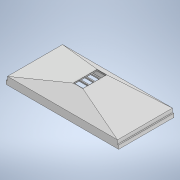
# Autodesk Inventor part: lejek
Saved by Autodesk Inventor 2020.3 (Build 243373000, 373)
## iProperties
Created: 2021-01-13
Part Number: lejek
Material: Ogólny
Document SubType Name: Modeling
Designer: sitar
Density: 1 g/cm^3
Appearance: Domyślna
Author: sitar
Autodesk Inventor part; units mm, degrees
ref_plane "YZ Plane" through (0, 0, 0) normal (1, 0, 0) x (0, 1, 0)
ref_plane "XY Plane" through (0, 0, 0) normal (0, 0, 1) x (1, 0, 0)
sketch "Szkic1" plane through (0, 0, 0) normal (0, 1, 0) x (-1, 0, 0)
  line L0 (57.6, -28.8) -> (-57.6, -28.8)
  line L1 (-57.6, -28.8) -> (-57.6, 28.8)
  line L2 (-57.6, 28.8) -> (57.6, 28.8)
  line L3 (57.6, 28.8) -> (57.6, -28.8)
  line L4 (57.6, -28.8) -> (-57.6, 28.8) construction
  line L5 (-57.6, -28.8) -> (57.6, 28.8) construction
  point P0 (0, 0)
  dimension "d0" = 115.2
  dimension "d1" = 57.6
  constraints: 12 end point, 2 midpoint, 2 parallel, 1 horizontal, 1 perpendicular
  measures "d0" distance of L1.end L2.end
  measures "d1" distance of L0.end L1.end
ref_plane "Płaszczyzna konstrukcyjna3" through (0, 12, 0) normal (0, 1, 0) x (-1, 0, 0)
sketch "Szkic11" plane through (0, 12, 0) normal (0, 1, 0) x (-1, 0, 0)
  line L0 (-5, -12.5) -> (5, -12.5)
  line L1 (5, -12.5) -> (5, 12.5)
  line L2 (5, 12.5) -> (-5, 12.5)
  line L3 (-5, 12.5) -> (-5, -12.5)
  line L4 (-5, -12.5) -> (5, 12.5) construction
  line L5 (5, -12.5) -> (-5, 12.5) construction
  point P0 (0, 0)
  dimension "d41" = 10
  dimension "d42" = 25
  constraints: 12 end point, 2 midpoint, 2 parallel, 1 horizontal, 1 perpendicular
  measures "d41" distance of L2.end L1.end
  measures "d42" distance of L1.end L0.end
loft "Wyciągnięcie złożone3" add profiles "Szkic11", "Szkic1"
shell "Skorupa3" thickness 1.2 removed faces 1 at (-19.2, 0, 9.6)
sketch "Szkic12" plane through (-4.8649, 10.8, -12.1059) normal (0, -1, 0) x (1, 0, 0)
  line L0 (0, 0) -> (0, 24.2118) projected
  line L1 (9.7297, 0) -> (57.0697, -14.67) projected
  line L2 (0, 24.2118) -> (9.7297, 24.2118)
  line L3 (9.7297, 24.2118) -> (9.7297, 0)
  line L4 (9.7297, 0) -> (0, 0)
  line L5 (0, 0) -> (0, 24.2118)
  point P0 (4.8649, 12.1059)
  constraints: 8 end point, 2 parallel, 1 horizontal, 1 perpendicular
extrude "Wyciągnięcie proste7" cut sketch "Szkic12" against normal blind 10
sketch "Szkic13" plane through (-57.6, 0, -28.8) normal (0, -1, 0) x (1, 0, 0)
  line L0 (115.2, 57.6) -> (115.2, 0) projected
  line L1 (52.6, 16.3) -> (0, 0) projected
  line L2 (115.2, 57.6) -> (0, 57.6)
  line L3 (0, 57.6) -> (0, 0)
  line L4 (0, 0) -> (115.2, 0)
  line L5 (115.2, 0) -> (115.2, 57.6)
  line L6 (5.3951, 55.5759) -> (109.8049, 55.5759) projected
  line L7 (109.8049, 2.0241) -> (5.3951, 2.0241) projected
  line L8 (109.8049, 55.5759) -> (5.3951, 55.5759)
  line L9 (5.3951, 55.5759) -> (5.3951, 2.0241)
  line L10 (5.3951, 2.0241) -> (109.8049, 2.0241)
  line L11 (109.8049, 2.0241) -> (109.8049, 55.5759)
  point P0 (57.6, 28.8)
  constraints: 16 end point, 4 parallel, 2 horizontal, 2 perpendicular
extrude "Wyciągnięcie proste8" add sketch "Szkic13" along normal blind 8
sketch "Szkic14" plane through (-57.6, -8, -28.8) normal (0, -1, 0) x (1, 0, 0)
  line L0 (115.2, 57.6) -> (0, 57.6) projected
  line L1 (115.2, 0) -> (0, 0)
  line L2 (0, 0) -> (0, 57.6)
  line L3 (0, 57.6) -> (115.2, 57.6)
  line L4 (115.2, 57.6) -> (115.2, 0)
  line L5 (115.2, 0) -> (0, 57.6) construction
  line L6 (0, 0) -> (115.2, 57.6) construction
  line L7 (116.4, 0) -> (-1.2, 0)
  line L8 (-1.2, 0) -> (-1.2, 57.6)
  line L9 (-1.2, 57.6) -> (116.4, 57.6)
  line L10 (116.4, 57.6) -> (116.4, 0)
  line L11 (116.4, 0) -> (-1.2, 57.6) construction
  line L12 (-1.2, 0) -> (116.4, 57.6) construction
  point P0 (57.6, 28.8)
  dimension "d52" = 117.6
  constraints: 24 end point, 4 midpoint, 4 parallel, 2 horizontal, 2 perpendicular
  measures "d52" distance of L8.end L9.end
extrude "Wyciągnięcie proste9" add sketch "Szkic14" against normal blind 4 contours L9 L10 L7 L4 | L2 L7 L8 L9
sketch "Szkic15" plane through (-5, 12, -12.5) normal (0, 1, 0) x (1, 0, 0)
  line L0 (9.8649, -24.6059) -> (9.8649, -0.3941) projected
  line L1 (0.1351, -13.1) -> (9.8649, -13.1)
  line L2 (9.8649, -13.1) -> (9.8649, -11.9)
  line L3 (9.8649, -11.9) -> (0.1351, -11.9)
  line L4 (0.1351, -11.9) -> (0.1351, -13.1)
  line L5 (0.1351, -13.1) -> (9.8649, -11.9) construction
  line L6 (9.8649, -13.1) -> (0.1351, -11.9) construction
  point P0 (5, -12.5)
  dimension "d55" = 1.2
  constraints: 12 end point, 2 midpoint, 2 parallel, 1 horizontal, 1 perpendicular, 1 point on line
  measures "d55" distance of L2.end L1.end
extrude "Wyciągnięcie proste10" add sketch "Szkic15" against normal blind 1.2
pattern_linear "Szyk prostokątny3" count 2 spacing 6 along (0, 0, -1) of "Wyciągnięcie proste10"
pattern_linear "Szyk prostokątny4" count 2 spacing 6 along (0, 0, 1) of "Wyciągnięcie proste10"
